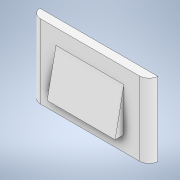
# Autodesk Inventor part: 스위치
Saved by Autodesk Inventor 2022 (Build 260153000, 153)
## iProperties
Created: 2022-10-26
Part Number: 스위치
Material: 일반
Document SubType Name: Modeling
Designer: whdls
Density: 1 g/cm^3
Appearance: 기본값
Author: whdls
Autodesk Inventor part; units mm, degrees
ref_plane "YZ Plane" through (0, 0, 0) normal (1, 0, 0) x (0, 1, 0)
ref_plane "XZ Plane" through (0, 0, 0) normal (0, 1, 0) x (-1, 0, 0)
sketch "스케치1" plane through (0, 0, 0) normal (0, 0, 1) x (1, 0, 0)
  line L0 (0, 0) -> (120, 0)
  line L1 (120, 0) -> (120, 75)
  line L2 (120, 75) -> (0, 75)
  line L3 (0, 75) -> (0, 0)
  dimension "d0" = 120
  dimension "d1" = 75
  constraints: 8 end point, 2 parallel, 1 horizontal, 1 perpendicular
  measures "d0" distance of L1.end L2.end
  measures "d1" distance of L0.end L1.end
extrude "돌출1" add sketch "스케치1" along normal blind 9
sketch "스케치2" plane through (0, 0, 9) normal (0, 0, 1) x (1, 0, 0)
  line L0 (25.5, 59.5) -> (94.5, 59.5)
  line L1 (94.5, 59.5) -> (94.5, 15.5)
  line L2 (94.5, 15.5) -> (25.5, 15.5)
  line L3 (25.5, 15.5) -> (25.5, 59.5)
  line L4 (0, 75) -> (0, 0) projected
  line L5 (0, 0) -> (120, 0) projected
  dimension "d4" = 44
  dimension "d5" = 69
  dimension "d6" = 25.5
  dimension "d7" = 15.5
  constraints: 8 end point, 2 parallel, 1 horizontal, 1 perpendicular
  measures "d4" distance of L0.end L1.end
  measures "d5" distance of L0.start L0.end
  measures "d6" distance between parallel lines of L4 L3
  measures "d7" distance between parallel lines of L5 L2
ref_plane "작업 평면1" through (94.5, 0, 0) normal (1, 0, 0) x (0, 0, -1)
sketch "스케치3" plane through (94.5, 0, 0) normal (1, 0, 0) x (0, 0, -1)
  line L0 (-9, 0) -> (-9, 75) projected
  line L1 (-9, 59.5) -> (-9, 15.5) projected
  line L2 (-9, 59.5) -> (-17.9999, 15.5)
  line L3 (-17.9999, 15.5) -> (-9, 15.5)
  point P0 (0, 0)
  dimension "d9" = 11.56
  dimension "d10" = 90
  constraints: 4 end point
  measures "d9" angle of L0 L2
  measures "d10" angle of L0 L3
extrude "돌출2" add sketch "스케치3" against normal blind 69
fillet "모깎기1" radius 10 1 edges at (120, 37.5, 9)
fillet "모깎기2" radius 10 1 edges at (0, 37.5, 9)
